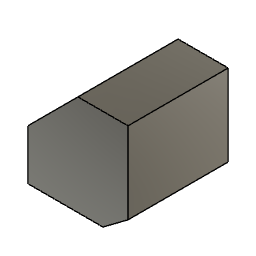
Suètone-drawing-object-01_02 v4 (Autodesk Fusion 360 design; units mm, degrees)
Autodesk Fusion 360 part; units mm, degrees
sketch "Esquisse1" plane through (0, 0, 0) normal (0, 0, 1) x (1, 0, 0)
  line L0 (40, 40) -> (-40, 40)
  line L1 (-40, 40) -> (-40, -40)
  line L2 (-40, -40) -> (40, -40)
  line L3 (40, -40) -> (40, 40)
  line L4 (40, 40) -> (-40, -40) construction
  line L5 (-40, 40) -> (40, -40) construction
  dimension "d1" = 80
  dimension "d2" = 80
  constraint horizontal L0
  constraint perpendicular L0 L1
  constraint parallel L0 L2
  constraint parallel L1 L3
  constraint coincident L4 origin
  constraint coincident L5 origin
  measures "d1" distance of L1.end L2.end
  measures "d2" distance of L0.end L1.end
extrude "Extrusion1" add sketch "Esquisse1" along normal blind 80 makes body 1
sketch "Esquisse2" plane through (0, -40, 0) normal (0, -1, 0) x (1, 0, 0)
  line L0 (-40, 0) -> (40, 0)
  line L1 (40, 0) -> (40, 80)
  line L2 (40, 80) -> (-40, 80)
  line L3 (-40, 80) -> (-40, 0)
  line L4 (0, 80) -> (-40, 40)
  constraint midpoint L2 L4.start
  constraint midpoint L3 L4.end
ref_plane "Plan de construction1" through (-20, -40, 60) normal (0.707107, 0, -0.707107) x (-0.707107, 0, -0.707107)
split "Scinder1" by plane through (-20, -40, 60) normal (0.707107, 0, -0.707107) bodies 1 makes body 2 at (40, -13.3333, 26.6667)
sketch "Esquisse3" plane through (-40, 0, 40) normal (-0.707107, 0, 0.707107) x (0, -1, 0)
  line L0 (40, 0) -> (40, 56.5685)
  line L1 (40, 56.5685) -> (-40, 56.5685)
  line L2 (-40, 56.5685) -> (-40, 0)
  line L3 (-40, 0) -> (40, 0)
  circle A0 centre (25, 30) radius 4
  circle A1 centre (8.3333, 30) radius 4
  circle A2 centre (-8.3333, 30) radius 4
  circle A3 centre (-25, 30) radius 4
  dimension "d8" = 8
  dimension "d11" = -50
  dimension "d12" = 0
  measures "d8" diameter of A0
sketch "Esquisse4" plane through (0, -40, 0) normal (0, -1, 0) x (1, 0, 0)
  line L0 (0, 80) -> (-40, 40)
  line L1 (-40, 40) -> (-40, 0)
  line L2 (-40, 0) -> (40, 0)
  line L3 (40, 0) -> (40, 80)
  line L4 (40, 80) -> (0, 80)
  line L5 (20, 0) -> (40, 15)
  constraint coincident L2 L5.start
  constraint coincident L3 L5.end
ref_plane "Plan de construction2" through (30, -40, 7.5) normal (-0.6, 0, 0.8) x (0.8, 0, 0.6)
split "Scinder2" by plane through (30, -40, 7.5) normal (-0.6, 0, 0.8) bodies 2 makes body 3 at (-6.6667, 40, 40)
delete_body "RemoveBody1" bodies 2
delete_body "RemoveBody2" bodies 1
extrude "Extrusion2" cut sketch "Esquisse3" against normal blind 90 contours A0 | A1 | A2 | A3 bodies 3
sketch "Esquisse5" plane through (0, 0, 0) normal (0, 0, -1) x (1, 0, 0)
  line L0 (20, -40) -> (20, 40)
  line L1 (20, 40) -> (-40, 40)
  line L2 (-40, 40) -> (-40, -40)
  line L3 (-40, -40) -> (20, -40)
  line L4 (-35, 35) -> (-31, 35)
  line L5 (-31, 35) -> (-31, -35)
  line L6 (-31, -35) -> (-35, -35)
  line L7 (-35, -35) -> (-35, 35)
  line L8 (-40, -40) -> (-40, 40)
  line L9 (-40, 0) -> (-35, 0)
  line L10 (15, -35) -> (11, -35)
  line L11 (11, -35) -> (11, 35)
  line L12 (11, 35) -> (15, 35)
  line L13 (15, 35) -> (15, -35)
  dimension "d18" = 70
  dimension "d19" = 5
  dimension "d22" = 4
  constraint horizontal L4
  constraint vertical L5
  constraint horizontal L6
  constraint vertical L7
  constraint midpoint L8 L9.start
  constraint coincident L7 L9.end
  constraint perpendicular L7 L9
  constraint midpoint L7 L9.end
  constraint horizontal L10
  constraint vertical L11
  constraint horizontal L12
  constraint vertical L13
  measures "d18" distance of L4.start L6.end
  measures "d19" distance of L2 L7
  measures "d22" distance of L10.start L10.end
extrude "Extrusion3" add sketch "Esquisse5" along normal blind 3 contours L4 L5 L6 L7 bodies 3
extrude "Extrusion4" add sketch "Esquisse5" along normal blind 3 contours L10 L11 L12 L13 bodies 3
